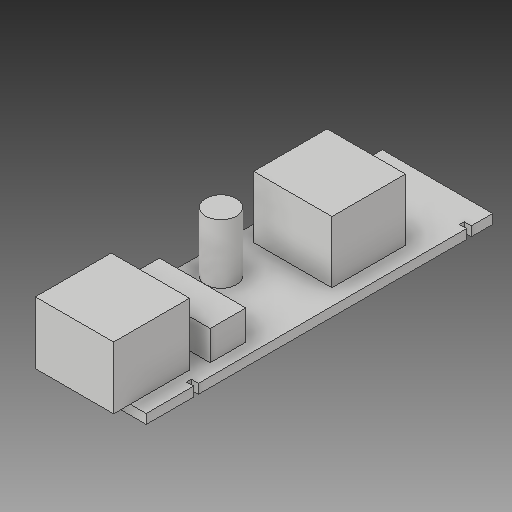
# Autodesk Inventor part: More powerful POE Splitter
Saved by Autodesk Inventor 2018 (Build 220112000, 112)
## iProperties
Created: 2019-09-20
Part Number: More powerful POE Splitter
Material: Generic
Document SubType Name: Modeling
Designer: Jacob
Density: 1 g/cm^3
Appearance: Default
Mass: 11.434 g
Surface Area: 61.6712 cm^2
Volume: 11.434 cm^3
Author: Jacob
Autodesk Inventor part; units mm, degrees
ref_plane "YZ Plane" through (0, 0, 0) normal (1, 0, 0) x (0, 1, 0)
ref_plane "XZ Plane" through (0, 0, 0) normal (0, 1, 0) x (-1, 0, 0)
ref_plane "XY Plane" through (0, 0, 0) normal (0, 0, 1) x (1, 0, 0)
sketch "Sketch1" plane through (0, 0, 0) normal (0, 1, 0) x (-1, 0, 0)
  line L0 (11.625, 36.5) -> (-11.625, 36.5)
  line L1 (-11.625, 36.5) -> (-11.625, -36.5)
  line L2 (-11.625, -36.5) -> (11.625, -36.5)
  line L3 (11.625, -36.5) -> (11.625, 36.5)
  line L4 (11.625, 36.5) -> (-11.625, -36.5) construction
  line L5 (-11.625, 36.5) -> (11.625, -36.5) construction
  point P0 (0, 0)
  dimension "d0" = 73
  dimension "d1" = 23.25
  constraints: 12 end point, 2 midpoint, 2 parallel, 1 horizontal, 1 perpendicular
  measures "d0" distance of L2.end L0.start
  measures "d1" distance of L1.end L2.end
extrude "Extrusion1" add sketch "Sketch1" along normal blind 2
sketch "Sketch2" plane through (0, 2, 0) normal (0, 1, 0) x (1, 0, 0)
  line L0 (-11.625, -36.5) -> (11.625, -36.5) projected
  line L1 (0, -36.5) -> (0, 36.5)
  line L2 (11.625, 36.5) -> (-11.625, 36.5) projected
  line L3 (-8.25, -40) -> (8.25, -40)
  line L4 (8.25, -40) -> (8.25, -24)
  line L5 (8.25, -24) -> (-8.25, -24)
  line L6 (-8.25, -24) -> (-8.25, -40)
  line L7 (-8.25, -40) -> (8.25, -24) construction
  line L8 (8.25, -40) -> (-8.25, -24) construction
  point P0 (0, 0)
  point P1 (0, -32)
  dimension "d4" = 3.5
  dimension "d5" = 16.5
  dimension "d6" = 16
  constraints: 14 end point, 4 midpoint, 2 parallel, 1 horizontal, 1 perpendicular, 1 point on line
  measures "d4" distance between parallel lines of L0 L3
  measures "d5" distance of L3.start L3.end
  measures "d6" distance of L3.end L4.end
extrude "Extrusion2" add sketch "Sketch2" along normal blind 13.1
sketch "Sketch3" plane through (0, 2, 0) normal (0, 1, 0) x (1, 0, 0)
  line L0 (-8.25, -24) -> (8.25, -24) projected
  line L1 (0, -24) -> (0, 36.5)
  line L2 (11.625, 36.5) -> (-11.625, 36.5) projected
  line L3 (-8.25, 6) -> (8.25, 6)
  line L4 (8.25, 6) -> (8.25, 21.5)
  line L5 (8.25, 21.5) -> (-8.25, 21.5)
  line L6 (-8.25, 21.5) -> (-8.25, 6)
  line L7 (-8.25, 6) -> (8.25, 21.5) construction
  line L8 (8.25, 6) -> (-8.25, 21.5) construction
  point P0 (0, 0)
  point P1 (0, 13.75)
  dimension "d9" = 15.5
  dimension "d10" = 16.5
  dimension "d11" = 15
  constraints: 14 end point, 4 midpoint, 2 parallel, 1 horizontal, 1 perpendicular, 1 point on line
  measures "d9" distance of L5.end L3.start
  measures "d10" distance of L4.end L5.end
  measures "d11" distance between parallel lines of L2 L5
extrude "Extrusion3" add sketch "Sketch3" along normal blind 13
sketch "Sketch4" plane through (0, 2, 0) normal (0, 1, 0) x (1, 0, 0)
  line L0 (8.25, 6) -> (-8.25, 6) projected
  line L1 (0, 6) -> (0, -24) construction
  line L2 (-8.25, -24) -> (8.25, -24) projected
  line L3 (-11.625, 36.5) -> (-11.625, -36.5) projected
  line L4 (-11.625, -3.5) -> (0, -3.5) construction
  line L5 (11.625, 36.5) -> (-11.625, 36.5) projected
  line L6 (-5.625, 36.5) -> (-5.625, -36.5) construction
  circle A0 centre (-5.625, -3.5) radius 3.25
  point P0 (0, 0)
  dimension "d14" = 9.5
  dimension "d15" = 6
  dimension "d16" = 6.5
  constraints: 6 end point, 5 point on line, 2 midpoint, 1 centre point, 1 perpendicular, 1 vertical
  measures "d14" distance between parallel lines of L0 L4
  measures "d15" distance between parallel lines of L3 L6
  measures "d16" diameter of A0
extrude "Extrusion4" add sketch "Sketch4" along normal blind 12.5
sketch "Sketch5" plane through (0, 2, 0) normal (0, 1, 0) x (1, 0, 0)
  line L0 (-9.1046, -20.5) -> (9.1046, -20.5)
  line L1 (9.1046, -20.5) -> (9.1046, -13)
  line L2 (9.1046, -13) -> (-9.1046, -13)
  line L3 (-9.1046, -13) -> (-9.1046, -20.5)
  line L4 (-9.1046, -20.5) -> (9.1046, -13) construction
  line L5 (9.1046, -20.5) -> (-9.1046, -13) construction
  line L6 (8.25, -24) -> (-8.25, -24) projected
  point P0 (0, 0)
  point P1 (0, -16.75)
  dimension "d19" = 7.5
  dimension "d20" = 18.2091
  dimension "d21" = 3.5
  constraints: 12 end point, 2 midpoint, 2 parallel, 1 horizontal, 1 perpendicular
  measures "d19" distance of L2.end L0.start
  measures "d20" distance of L0.start L0.end
  measures "d21" distance between parallel lines of L6 L0
extrude "Extrusion5" add sketch "Sketch5" along normal blind 6.25
sketch "Sketch6" plane through (0, 2, 0) normal (0, 1, 0) x (1, 0, 0)
  line L0 (-11.9415, 31.5) -> (11.625, 31.5) construction
  line L1 (11.625, -36.5) -> (11.625, 36.5) projected
  line L2 (-11.625, 36.5) -> (-11.625, -36.5) projected
  line L3 (-11.625, -26) -> (11.625, -26) construction
  line L4 (11.625, 36.5) -> (-11.625, 36.5) projected
  line L5 (-11.625, 31) -> (-10.125, 31)
  line L6 (-10.125, 31) -> (-10.125, 32)
  line L7 (-10.125, 32) -> (-11.625, 32)
  line L8 (-11.625, 32) -> (-11.625, 31)
  line L9 (-11.625, 31) -> (-10.125, 32) construction
  line L10 (-10.125, 31) -> (-11.625, 32) construction
  line L11 (10.125, 31) -> (11.625, 31)
  line L12 (11.625, 31) -> (11.625, 32)
  line L13 (11.625, 32) -> (10.125, 32)
  line L14 (10.125, 32) -> (10.125, 31)
  line L15 (10.125, 31) -> (11.625, 32) construction
  line L16 (11.625, 31) -> (10.125, 32) construction
  line L17 (-11.625, -26.5) -> (-10.125, -26.5)
  line L18 (-10.125, -26.5) -> (-10.125, -25.5)
  line L19 (-10.125, -25.5) -> (-11.625, -25.5)
  line L20 (-11.625, -25.5) -> (-11.625, -26.5)
  line L21 (-11.625, -26.5) -> (-10.125, -25.5) construction
  line L22 (-10.125, -26.5) -> (-11.625, -25.5) construction
  line L23 (10.125, -26.5) -> (11.625, -26.5)
  line L24 (11.625, -26.5) -> (11.625, -25.5)
  line L25 (11.625, -25.5) -> (10.125, -25.5)
  line L26 (10.125, -25.5) -> (10.125, -26.5)
  line L27 (10.125, -26.5) -> (11.625, -25.5) construction
  line L28 (11.625, -26.5) -> (10.125, -25.5) construction
  point P0 (0, 0)
  point P1 (-10.875, 31.5)
  point P2 (10.875, 31.5)
  point P3 (-10.875, -26)
  point P4 (10.875, -26)
  dimension "d24" = 57.5
  dimension "d25" = 5
  dimension "d26" = 1
  dimension "d27" = 1.5
  dimension "d28" = 0
  dimension "d29" = 1
  dimension "d30" = 1.5
  dimension "d31" = 0
  dimension "d32" = 0
  dimension "d33" = 1.5
  dimension "d34" = 1
  dimension "d35" = 0
  dimension "d36" = 1.5
  dimension "d37" = 1
  constraints: 52 end point, 8 midpoint, 8 parallel, 7 point on line, 6 horizontal, 4 perpendicular
  measures "d24" distance between parallel lines of L0 L3
  measures "d25" distance between parallel lines of L4 L0
  measures "d26" distance of L5.end L6.end
  measures "d27" distance of L6.end L7.end
  measures "d28" distance between parallel lines of L2 L8
  measures "d29" distance of L13.end L11.start
  measures "d30" distance of L12.end L13.end
  measures "d31" distance between parallel lines of L1 L12
  measures "d32" distance between parallel lines of L1 L24
  measures "d33" distance of L24.end L25.end
  measures "d34" distance of L25.end L23.start
  measures "d35" distance between parallel lines of L2 L20
  measures "d36" distance of L17.start L17.end
  measures "d37" distance of L17.end L18.end
extrude "Extrusion6" cut sketch "Sketch6" against normal blind 6.25
body "Solid1"
